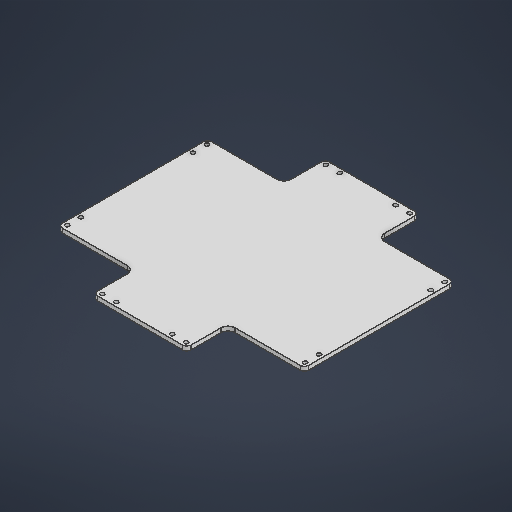
# Autodesk Inventor part: cover
Saved by Autodesk Inventor 2026.1 (Build 301233000, 233)
## iProperties
Created: 2026-03-31
Part Number: cover
Material: Generic
Document SubType Name: Modeling
Designer: emanuel
Density: 1 g/cm^3
Appearance: Default
Author: emanuel
Autodesk Inventor part; units mm, degrees
ref_plane "YZ Plane" through (0, 0, 0) normal (1, 0, 0) x (0, 1, 0)
ref_plane "XZ Plane" through (0, 0, 0) normal (0, 1, 0) x (-1, 0, 0)
ref_plane "XY Plane" through (0, 0, 0) normal (0, 0, 1) x (1, 0, 0)
sketch "Sketch1" plane through (0, 0, 0) normal (0, 1, 0) x (-1, 0, 0)
  line L0 (-20, 80) -> (20, 80)
  line L1 (20, 80) -> (20, -80)
  line L2 (20, -80) -> (-20, -80)
  line L3 (-20, -80) -> (-20, 80)
  line L4 (-20, 80) -> (20, -80) construction
  line L5 (20, 80) -> (-20, -80) construction
  line L6 (20, 80) -> (30, 80)
  line L7 (30, 80) -> (30, -80)
  line L8 (30, -80) -> (20, -80)
  line L9 (20, -80) -> (20, 80)
  line L10 (-20, 80) -> (-30, 80)
  line L11 (-30, 80) -> (-30, -80)
  line L12 (-30, -80) -> (-20, -80)
  line L13 (-20, -80) -> (-20, 80)
  circle A0 centre (30, 80) radius 1.5
  circle A1 centre (20, 80) radius 1.5
  circle A2 centre (-20, 80) radius 1.5
  circle A3 centre (-30, 80) radius 1.5
  circle A4 centre (30, -80) radius 1.5
  circle A5 centre (-30, -80) radius 1.5
  line L14 (-85.15, 40) -> (85.15, 40)
  line L15 (85.15, 40) -> (85.15, -40)
  line L16 (85.15, -40) -> (-85.15, -40)
  line L17 (-85.15, -40) -> (-85.15, 40)
  line L18 (-85.15, 40) -> (85.15, -40) construction
  line L19 (85.15, 40) -> (-85.15, -40) construction
  line L20 (85.15, 40) -> (-85.15, 40)
  line L21 (-85.15, 40) -> (-85.15, 50)
  line L22 (-85.15, 50) -> (85.15, 50)
  line L23 (85.15, 50) -> (85.15, 40)
  line L24 (85.15, -40) -> (-85.15, -40)
  line L25 (-85.15, -40) -> (-85.15, -50)
  line L26 (-85.15, -50) -> (85.15, -50)
  line L27 (85.15, -50) -> (85.15, -40)
  circle A6 centre (-85.15, 50) radius 1.5
  circle A7 centre (-85.15, 40) radius 1.5
  circle A8 centre (-85.15, -40) radius 1.5
  circle A9 centre (-85.15, -50) radius 1.5
  circle A10 centre (-20, -80) radius 1.5
  circle A11 centre (20, -80) radius 1.5
  circle A12 centre (85.15, -40) radius 1.5
  circle A13 centre (85.15, -50) radius 1.5
  circle A14 centre (85.15, 50) radius 1.5
  circle A15 centre (85.15, 40.1297) radius 1.5
  line L28 (85.15, 50) -> (-85.15, 50)
  line L29 (-85.15, 50) -> (-85.15, 53.5)
  line L30 (-85.15, 53.5) -> (85.15, 53.5)
  line L31 (85.15, 53.5) -> (85.15, 50)
  line L32 (-30, 80) -> (-33.5, 80)
  line L33 (-33.5, 80) -> (-33.5, -80)
  line L34 (-33.5, -80) -> (-30, -80)
  line L35 (-30, -80) -> (-30, 80)
  line L36 (85.15, -50) -> (-85.15, -50)
  line L37 (-85.15, -50) -> (-85.15, -53.5)
  line L38 (-85.15, -53.5) -> (85.15, -53.5)
  line L39 (85.15, -53.5) -> (85.15, -50)
  line L40 (30, -80) -> (-33.5, -80)
  line L41 (-33.5, -80) -> (-33.5, -83)
  line L42 (-33.5, -83) -> (30, -83)
  line L43 (30, -83) -> (30, -80)
  line L44 (30, 80) -> (33.5, 80)
  line L45 (33.5, 80) -> (33.5, -83)
  line L46 (33.5, -83) -> (30, -83)
  line L47 (30, -83) -> (30, 80)
  line L48 (33.5, 80) -> (-33.5, 80)
  line L49 (-33.5, 80) -> (-33.5, 83)
  line L50 (-33.5, 83) -> (33.5, 83)
  line L51 (33.5, 83) -> (33.5, 80)
  line L52 (85.15, 53.5) -> (88.15, 53.5)
  line L53 (88.15, 53.5) -> (88.15, -53.5)
  line L54 (88.15, -53.5) -> (85.15, -53.5)
  line L55 (85.15, -53.5) -> (85.15, 53.5)
  line L56 (-85.15, 53.5) -> (-88.15, 53.5)
  line L57 (-88.15, 53.5) -> (-88.15, -53.5)
  line L58 (-88.15, -53.5) -> (-85.15, -53.5)
  line L59 (-85.15, -53.5) -> (-85.15, 53.5)
  point P0 (0, 0)
  point P1 (-33.5, 53.5)
  point P2 (-33.5, -53.5)
  point P3 (33.5, -53.5)
  point P4 (33.5, 53.5)
  point P5 (-18.5, 80)
  point P6 (-20, 78.5)
  point P7 (20, 78.5)
  point P8 (18.5, 80)
  dimension "d0" = 40
  dimension "d1" = 160
  dimension "d2" = 10
  dimension "d3" = 10
  dimension "d4" = 3
  dimension "d5" = 3
  dimension "d6" = 3
  dimension "d7" = 3
  dimension "d8" = 3
  dimension "d9" = 3
  dimension "d10" = 170.3
  dimension "d11" = 80
  dimension "d12" = 10
  dimension "d13" = 10
  dimension "d14" = 3
  dimension "d15" = 3
  dimension "d16" = 3
  dimension "d17" = 3
  dimension "d18" = 3
  dimension "d19" = 3
  dimension "d20" = 3
  dimension "d21" = 3
  dimension "d22" = 3
  dimension "d23" = 3
  dimension "d24" = 3.5
  dimension "d25" = 3.5
  dimension "d26" = 3.5
  dimension "d27" = 3
  dimension "d28" = 3.5
  dimension "d29" = 3
  dimension "d30" = 3
  dimension "d31" = 3
  constraints: 120 end point, 28 parallel, 16 centre point, 15 coincident, 14 horizontal, 14 perpendicular, 5 point on line, 4 midpoint
  measures "d0" distance of L1.end L2.end
  measures "d1" distance of L0.end L1.end
  measures "d2" distance of L7.end L8.end
  measures "d3" distance of L12.end L11.end
  measures "d4" diameter of A0
  measures "d5" diameter of A1
  measures "d6" diameter of A2
  measures "d7" diameter of A3
  measures "d8" diameter of A4
  measures "d9" diameter of A5
  measures "d10" distance of L15.end L16.end
  measures "d11" distance of L14.end L15.end
  measures "d12" distance of L20.end L21.end
  measures "d13" distance of L25.end L24.end
  measures "d14" diameter of A6
  measures "d15" diameter of A7
  measures "d16" diameter of A8
  measures "d17" diameter of A9
  measures "d18" diameter of A10
  measures "d19" diameter of A11
  measures "d20" diameter of A12
  measures "d21" diameter of A13
  measures "d22" diameter of A14
  measures "d23" diameter of A15
  measures "d24" distance of L28.end L29.end
  measures "d25" distance of L34.end L33.end
  measures "d26" distance of L37.end L36.end
  measures "d27" distance of L41.end L40.end
  measures "d28" distance of L45.end L46.end
  measures "d29" distance of L48.end L49.end
  measures "d30" distance of L53.end L54.end
  measures "d31" distance of L58.end L57.end
extrude "Extrusion1" add sketch "Sketch1" along normal blind 3 contours A2 L10 A3 L32 L49 L50 L51 L44 A0 L6 A1 L0 | L0 A1 L1 L30 L3 A2 | L3 L30 L11 A3 L10 A2 | L30 L1 L22 L3 | L3 L22 L11 L30 | L6 A0 L7 L30 L1 A1 | L22 L1 L14 L3 | L3 L14 L11 L22 | L30 L33 L32 A3 L11 | L11 L22 L33 L30 | L30 L7 L22 L1 | L14 L1 L16 L3 | L3 L16 L11 L14 | L11 L14 L33 L22 | L22 L7 L14 L1 | L33 L22 A6 L29 L30 | L30 L45 L22 L7 | L7 A0 L44 L45 L30 | L16 L1 L26 L3 | L3 L26 L11 L16 | L11 L16 L33 L14 | L14 L7 L16 L1 | L33 L14 A7 L21 A6 L22 | L22 L45 L14 L7 | L29 A6 L21 A7 L17 A8 L25 A9 L37 L58 L57 L56 | L30 L31 A14 L22 L45 | L26 L1 L38 L3 | L3 L38 L11 L26 | L16 L7 L26 L1 | L11 L26 L33 L16 | L33 L16 A8 L17 A7 L14 | L14 L45 L16 L7 | L22 A14 L23 A15 L14 L45 | L52 L53 L54 L39 A13 L27 A12 L15 A15 L23 A14 L31 | L38 L1 A11 L2 A10 L3 | L3 A10 L12 A5 L11 L38 | L11 L38 L33 L26 | L26 L7 L38 L1 | L16 L45 L26 L7 | L33 L26 A9 L25 A8 L16 | L14 A15 L15 A12 L16 L45 | L11 A5 L34 L33 L38 | L38 L7 A4 L8 A11 L1 | L33 L38 L37 A9 L26 | L26 L45 L38 L7 | L16 A12 L27 A13 L26 L45 | L2 A11 L8 A4 L43 L42 L41 L34 A5 L12 A10 | L38 L45 L46 L43 A4 L7 | L26 A13 L39 L38 L45
fillet "Fillet1" radius 5 4 edges at (33.5, 1.5, 53.5) (-33.5, 1.5, 53.5) (-33.5, 1.5, -53.5) (33.5, 1.5, -53.5)
fillet "Fillet2" radius 3 8 edges at (-88.15, 1.5, 53.5) (-88.15, 1.5, -53.5) (-33.5, 1.5, -83) (33.5, 1.5, -83) (88.15, 1.5, -53.5) (88.15, 1.5, 53.5) (33.5, 1.5, 83) (-33.5, 1.5, 83)
body "Solid1"
